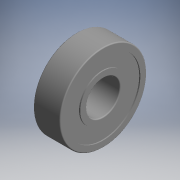
# Autodesk Inventor part: B6000ZZ
Saved by Autodesk Inventor 2017.3 (Build 213256000, 256)
## iProperties
Part Number: B6000ZZ
Material: Generic
Catalog Web Link: www.cadenas.de
Description: B6_ _ _ZZ, SB6_ _ _ZZ-Deep Groove Ball Bearings - Double Shield Type
Vendor: MISUMI
Document SubType Name: Modeling
Designer: partserver
Manufacturer: MISUMI
Mass: 3.45896 g
Surface Area: 18.5551 cm^2
Volume: 3.45896 cm^3
Density: 1 g/cm^3
Appearance: PSOLRGB-175-175-175
Category: PARTsolutions
Company: MISUMI
Title: B6000ZZ
Author: Cadenas PARTsolutions
Comments: Deep Groove Ball Bearings - Double Shield Type
PSOL_IDENT_0: {$CADENAS_DATA\23d-libs\misumi\metric\12_bearing_holders\sb6010zz.prj},171 {VTYP=3D},{NB=B6000ZZ},{L
PSOL_IDENT_1: INA=B6000ZZ},{NN=B6_ _ _ZZ, SB6_ _ _ZZ},{DATE=22.10.2019 07:39:52},{GEOMDATE=22.10.2019 06:26:04},{V
PSOL_IDENT_2: ERSION=},{LINEID=40},{WBVAR=TS},{WBNUMERIC=}  {NB=B6000ZZ},{LINA=B6000ZZ},{KT=DUMMY},{PN=B6000ZZ},{T
PSOL_IDENT_3: S=},{TS1= '', 'Steel', 'S', 'Stainless Steel'},{MAT=52100 Bearing Steel},{BN=6000ZZ},{DD=10},{D=26},
PSOL_IDENT_4: {B=8},{RR=0.3},{CR=4.55},{COR=1.96},{CRS=4.55},{CRSS=3.87},{CORS=1.96},{CORSS=1.58},{DD1=24.50},{R1=
PSOL_IDENT_5: 0.20},{R2=0.3},{DSMIN=12.0},{DSMAX=13.50},{DS1=13.50},{DDHH=24.0},{R=0.3},{MASS=19},{MASS11=19},{AA=
PSOL_IDENT_6: 7.3380},{BB=1.9000},{CC=1.9500},{TYS=w/o Retaining Ring}
NB: B6000ZZ
NN: B6_ _ _ZZ, SB6_ _ _ZZ
NT: Deep Groove Ball Bearings - Double Shield Type
NBSYN: $PN.
LINA: B6000ZZ
CATALOG: Misumi
PN: B6000ZZ
TS: Steel
MAT: 52100 Bearing Steel
BN: 6000ZZ
DD: 10
D: 26
B: 8
RR: 0.3
CR: 4.55
COR: 1.96
DSMIN: 12
DSMAX: 13.5
DDHH: 24
R: 0.3
MASS: 19
SUPPLIER: MISUMI
ARTICLENO: B6000ZZ
BOMINFO: B6000ZZ
CREATOR: CADENAS GmbH
Autodesk Inventor part; units mm, degrees
sketch "Sketch_1" plane through (0, 0, 0) normal (0, 0, 1) x (1, 0, 0)
  line L0 (8, 0) -> (0, 0)
  arc A0 (0, 5.3) -> (0.3, 5) centre (0.3, 5.3) ccw
  line L1 (0.3, 5) -> (7.7, 5)
  arc A1 (7.7, 5) -> (8, 5.3) centre (7.7, 5.3) ccw
  line L2 (8, 5.3) -> (8, 6.95)
  line L3 (8, 6.95) -> (7.669, 6.95)
  line L4 (7.669, 6.95) -> (7.669, 11.1)
  line L5 (7.669, 11.1) -> (8, 11.1)
  line L6 (8, 11.1) -> (8, 12.7)
  arc A2 (8, 12.7) -> (7.7, 13) centre (7.7, 12.7) ccw
  line L7 (7.7, 13) -> (0.3, 13)
  arc A3 (0.3, 13) -> (0, 12.7) centre (0.3, 12.7) ccw
  line L8 (0, 12.7) -> (0, 11.1)
  line L9 (0, 11.1) -> (0.331, 11.1)
  line L10 (0.331, 11.1) -> (0.331, 6.95)
  line L11 (0.331, 6.95) -> (0, 6.95)
  line L12 (0, 6.95) -> (0, 5.3)
  constraints: 26 end point, 8 point on circle, 4 centre point
revolve "Revolution1" add sketch "Sketch_1" angle 360 about axis through (8, 0, 0) along (1, 0, 0)
ref_plane "center_point_XY" through (4, 0, 0) normal (1, 0, 0) x (0, 0, -1)
ref_plane "center_point_YZ" through (4, 0, 0) normal (0, 0, -1) x (0, 1, 0)
ref_plane "center_point_ZX" through (4, 0, 0) normal (0, 1, 0) x (1, 0, 0)
ref_plane "to_housing_XY" through (0, 0, 0) normal (1, 0, 0) x (0, 0, -1)
ref_plane "to_housing_YZ" through (0, 0, 0) normal (0, 0, -1) x (0, 1, 0)
ref_plane "to_housing_ZX" through (0, 0, 0) normal (0, 1, 0) x (1, 0, 0)
ref_plane "to_ring_XY" through (7.338, 0, 0) normal (1, 0, 0) x (0, 0, -1)
ref_plane "to_ring_YZ" through (7.338, 0, 0) normal (0, 0, -1) x (0, 1, 0)
ref_plane "to_ring_ZX" through (7.338, 0, 0) normal (0, 1, 0) x (1, 0, 0)
body "Solid1"
